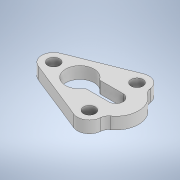
# Autodesk Inventor part: Part4
Saved by Autodesk Inventor 2021 (Build 250183000, 183)
## iProperties
Created: 2022-04-24
Part Number: Part4
Material: Generic
Document SubType Name: Modeling
Designer: hp
Density: 1 g/cm^3
Appearance: Default
Author: hp
Autodesk Inventor part; units mm, degrees
ref_plane "YZ Plane" through (0, 0, 0) normal (1, 0, 0) x (0, 1, 0)
ref_plane "XZ Plane" through (0, 0, 0) normal (0, 1, 0) x (-1, 0, 0)
ref_plane "XY Plane" through (0, 0, 0) normal (0, 0, 1) x (1, 0, 0)
sketch "Sketch1" plane through (0, 0, 0) normal (0, 1, 0) x (-1, 0, 0)
  arc A0 (90.3834, -85.781) -> (90.3834, -67.2115) centre (86.6694, -76.4962) ccw
  arc A1 (40.3834, -47.2115) -> (26.6694, -56.4962) centre (36.6694, -56.4962) ccw
  arc A2 (26.6694, -96.4962) -> (40.3834, -105.781) centre (36.6694, -96.4962) ccw
  line L0 (40.3834, -47.2115) -> (90.3834, -67.2115)
  line L1 (90.3834, -85.781) -> (40.3834, -105.781)
  circle A3 centre (86.6694, -76.4962) radius 5
  circle A4 centre (36.6694, -56.4962) radius 5
  circle A5 centre (36.6694, -96.4962) radius 5
  arc A6 (54.9839, -83.5808) -> (54.6671, -69.8665) centre (64.6694, -76.4962) ccw
  arc A7 (34.6694, -70.7615) -> (34.6706, -82.7615) centre (34.6706, -76.7615) ccw
  line L2 (34.6694, -70.7615) -> (53.0001, -70.7615)
  line L3 (53.3697, -82.7615) -> (34.6706, -82.7615)
  arc A8 (23.7082, -61.243) -> (23.7082, -92.2801) centre (34.6706, -76.7615) ccw
  line L4 (26.6694, -96.4962) -> (26.6694, -97.9974)
  line L5 (26.6694, -55.5256) -> (26.6694, -56.4962)
  arc A9 (23.7082, -61.243) -> (26.6694, -55.5256) centre (19.6694, -55.5256) ccw
  arc A10 (26.6694, -97.9974) -> (23.7082, -92.2801) centre (19.6694, -97.9974) ccw
  arc A11 (53.0001, -70.7615) -> (54.6671, -69.8665) centre (53.0001, -68.7615) ccw
  arc A12 (54.9839, -83.5808) -> (53.3697, -82.7615) centre (53.3697, -84.7615) ccw
  point P0 (0, 0)
  point P1 (54.4349, -82.7615)
  point P2 (54.1284, -70.7615)
  point P3 (26.6694, -59.5284)
  point P4 (26.6694, -93.9947)
  dimension "d0" = 50
  dimension "d1" = 0
  dimension "d2" = 20
  dimension "d3" = 20
  dimension "d4" = 20
  dimension "d5" = 40
  dimension "d6" = 20
  dimension "d7" = 10
  dimension "d8" = 10
  dimension "d9" = 10
  dimension "d10" = 12
  dimension "d11" = 30
  dimension "d12" = 6
  dimension "d13" = 0
  dimension "d14" = 22
  dimension "d16" = 7
  dimension "d17" = 7
  dimension "d18" = 2
  constraints: 24 point on circle, 17 tangent, 13 centre point, 12 end point, 4 point on line, 3 coincident, 1 concentric, 1 equal radius, 1 horizontal, 1 parallel
  measures "d0" horizontal distance of A1.centre A0.centre
  measures "d1" horizontal distance of A1.centre A2.centre
  measures "d2" diameter of A2
  measures "d3" diameter of A1
  measures "d4" diameter of A0
  measures "d5" distance of A2.centre A1.centre
  measures "d6" vertical distance of A1.centre A0.centre
  measures "d7" diameter of A5
  measures "d8" diameter of A3
  measures "d9" diameter of A4
  measures "d10" radius of A6
  measures "d11" distance of A7.centre A6.centre
  measures "d12" radius of A7
  measures "d13" vertical distance of A0.centre A6.centre
  measures "d14" distance of A3.centre A6.centre
  measures "d16" radius of A9
  measures "d17" radius of A10
  measures "d18" radius of A11
extrude "Extrusion1" add sketch "Sketch1" along normal blind 10
equation "\"d3\" = d2"
equation "\"d4\" = d2"
equation "\"d6\" = 0.5 * d5"
equation "\"d8\" = d7"
equation "\"d9\" = d7"
body "Solid1"
